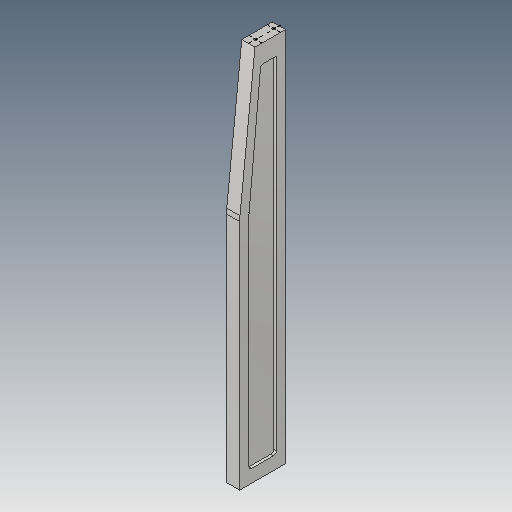
# Autodesk Inventor part: ZcolStiffer
Saved by Autodesk Inventor 2019 (Build 230136000, 136)
## iProperties
Created: 2018-10-03
Part Number: ZcolStiffer
Material: Aluminum 6061-AHC
Document SubType Name: Modeling
Designer: LillaHunden
Density: 2.7 g/cm^3
Appearance: Aluminum - Dark
Mass: 574.456 g
Surface Area: 583.617 cm^2
Volume: 212.761 cm^3
Author: LillaHunden
Autodesk Inventor part; units mm, degrees
ref_plane "YZ Plane" through (0, 0, 0) normal (1, 0, 0) x (0, 1, 0)
ref_plane "XZ Plane" through (0, 0, 0) normal (0, 1, 0) x (-1, 0, 0)
ref_plane "XY Plane" through (0, 0, 0) normal (0, 0, 1) x (1, 0, 0)
ref_plane "Work Plane1" through (0, 0, 0) normal (0, 0, 1) x (1, 0, 0)
sketch "Sketch1" plane through (0, 0, 0) normal (0, 0, 1) x (1, 0, 0)
  line L0 (33.6143, 326.2667) -> (51.0643, 326.2667) construction
  line L1 (35.1393, 326.2667) -> (49.5393, 326.2667)
  line L2 (49.5393, 326.2667) -> (49.5393, -83.7333)
  line L3 (49.5393, -83.7333) -> (35.1393, -83.7333)
  line L4 (35.1393, -83.7333) -> (35.1393, 326.2667)
  line L5 (34.6393, -83.7333) -> (19.9455, -83.7333) projected
  point P0 (42.3393, 326.2667)
  point P1 (42.3393, 326.2667)
  point P2 (42.3393, -83.7333)
  dimension "d0" = 14.4
  constraints: 8 end point, 3 midpoint, 2 parallel, 1 coincident, 1 horizontal, 1 horizontal alignment, 1 perpendicular, 1 point on line
  measures "d0" distance of L2.end L3.end
extrude "Extrusion1" add sketch "Sketch1" along normal blind 50
sketch "Sketch4" plane through (35.1393, -83.7333, 0) normal (-1, 0, 0) x (0, 0, 1)
  line L0 (0, 410) -> (50, 410) construction
  line L1 (0, 0) -> (0, 410) construction
  line L2 (0, 0) -> (50, 0) construction
  line L3 (50, 410) -> (50, 0) construction
  line L4 (40, 14) -> (10, 14)
  line L5 (27.0527, 390) -> (39.7039, 257.1374)
  line L6 (39.7039, 257.1374) -> (40, 254.1656)
  line L7 (40, 254.1656) -> (40, 14)
  line L8 (10, 390) -> (27.0527, 390)
  line L9 (5, 0) -> (-10, 0) construction
  line L10 (5, 0) -> (5, 410) construction
  line L11 (-10, 410) -> (5, 410) construction
  line L12 (-10, 0) -> (-10, 410) construction
  line L13 (10, 14) -> (10, 390)
  line L14 (0, 0) -> (0, 410) projected
  point P0 (0, 83.7333)
  point P1 (5, 390)
  dimension "d20" = 10
  dimension "d21" = 20
  dimension "d22" = 14
  dimension "d50" = 10
  constraints: 12 end point, 1 horizontal, 1 parallel, 1 point on line
  measures "d20" distance between parallel lines of L3 L7
  measures "d21" distance between parallel lines of L0 L8
  measures "d22" distance between parallel lines of L4 L2
  measures "d50" distance between parallel lines of L1 L13
extrude "Extrusion3" cut sketch "Sketch4" against normal blind 3
fillet "Fillet1" radius 3 3 edges at (36.6393, -69.7333, 10) (36.6393, -69.7333, 40) (36.6393, 306.2667, 27.0527)
ref_plane "Work Plane2" through (42.3393, -83.7333, 0) normal (-1, 0, 0) x (0, 0, 1)
mirror "Mirror2" about plane through (42.3393, -83.7333, 0) normal (-1, 0, 0) of "Extrusion3", "Fillet1"
sketch "Sketch6" plane through (49.5393, -83.7333, 0) normal (1, 0, 0) x (0, 0, -1)
  line L0 (-50, 410) -> (-50, 0) projected
  line L1 (-50, 256.2615) -> (-33.3099, 410)
  line L2 (0, 410) -> (-50, 410) projected
  point P0 (0, 83.7333)
  constraints: 2 end point, 2 point on line
extrude "Extrusion4" cut sketch "Sketch6" against normal through all
fillet "Fillet2" radius 50 1 edges at (42.3393, 172.5282, 50)
sketch "Sketch3" plane through (35.1393, 326.2667, 0) normal (0, 1, 0) x (1, 0, 0)
  point P0 (7.4895, -25.5)
  point P1 (7.4895, -5.5)
sketch "Sketch7" plane through (0, 0, 0) normal (0, 0, -1) x (-1, 0, 0)
  point P0 (-42.3393, 309.2667)
  point P1 (-42.3393, 284.2667)
  point P2 (-42.3393, 259.2667)
  point P3 (-42.3393, 234.2667)
  point P4 (-42.3393, 209.2667)
  point P5 (-42.3393, 184.2667)
  point P6 (-42.3393, 159.2667)
  point P7 (-42.3393, 134.2667)
  point P8 (-42.3393, 109.2667)
  point P9 (-42.3393, 84.2667)
  point P10 (-42.3393, 59.2667)
  point P11 (-42.3393, 34.2667)
  point P12 (-42.3393, 9.2667)
  point P13 (-42.3393, -15.7333)
  point P14 (-42.3393, -40.7333)
  point P15 (-42.3393, -65.7333)
hole "Hole4" at (42.3393, 309.2667, 0) at (42.3393, 284.2667, 0) at (42.3393, 259.2667, 0) at (42.3393, 234.2667, 0) at (42.3393, 209.2667, 0) at (42.3393, 184.2667, 0) at (42.3393, 159.2667, 0) at (42.3393, 134.2667, 0) at (42.3393, 109.2667, 0) at (42.3393, 84.2667, 0) at (42.3393, 59.2667, 0) at (42.3393, 34.2667, 0) at (42.3393, 9.2667, 0) at (42.3393, -15.7333, 0) at (42.3393, -40.7333, 0) at (42.3393, -65.7333, 0) direction (0, 0, 1) diameter 2.459 depth 11 tip angle 120 thread size "M3x0.5" class "6H" standard "ISO Metric profile"
sketch "Sketch8" plane through (35.1393, 326.2667, 0) normal (0, 1, 0) x (1, 0, 0)
  point P0 (7.1395, -5.5817)
  point P1 (7.1395, -25.5817)
hole "Hole5" at (42.2788, 326.2667, 5.5817) at (42.2788, 326.2667, 25.5817) direction (0, -1, 0) diameter 3.242 depth 10 tip angle 120 thread size "M4x0.7" class "6H" standard "ISO Metric profile"
sketch "Sketch9" plane through (35.1393, -83.7333, 0) normal (0, -1, 0) x (1, 0, 0)
  line L0 (0, 50) -> (14.4, 50) projected
  line L1 (7.2, 50) -> (7.2, 0) construction
  line L2 (14.4, 0) -> (0, 0) projected
  point P0 (-35.1393, 0)
  point P1 (7.2, 40)
  point P2 (7.2, 10)
  point P3 (7.2, 25)
  dimension "d51" = 10
  dimension "d52" = 10
  constraints: 3 midpoint, 2 end point, 2 point on line
  measures "d51" distance from line of L2 point (7.2, 10)
  measures "d52" distance from line of L0 point (7.2, 40)
hole "Hole7" at (42.3393, -83.7333, 40) at (42.3393, -83.7333, 25) at (42.3393, -83.7333, 10) direction (0, 1, 0) diameter 4.134 depth 14.2 thread size "M5x0.8" class "6H" standard "ISO Metric profile"
body "Solid1"
